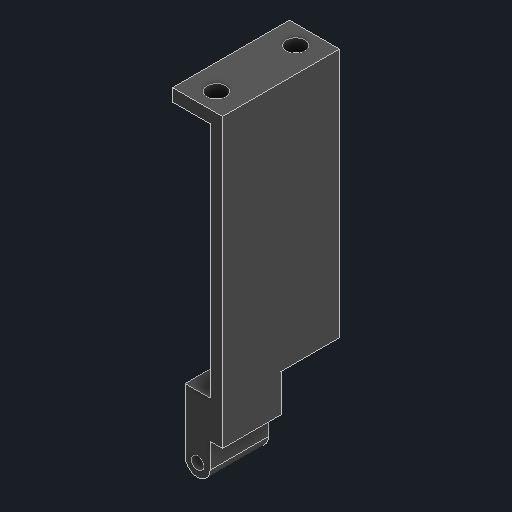
# Autodesk Inventor part: rudder_base
Saved by Autodesk Inventor 2022.2 (Build 262287010, 287A)
## iProperties
Created: 2022-03-30
Part Number: rudder_base
Material: Generic
Document SubType Name: Modeling
Designer: kardo
Density: 1 g/cm^3
Appearance: Dark Plastic
Author: kardo
Autodesk Inventor part; units mm, degrees
ref_plane "YZ Plane" through (0, 0, 0) normal (1, 0, 0) x (0, 1, 0)
ref_plane "XZ Plane" through (0, 0, 0) normal (0, 1, 0) x (-1, 0, 0)
ref_plane "XY Plane" through (0, 0, 0) normal (0, 0, 1) x (1, 0, 0)
derived "parameters_powertrain.ipt"
sketch "sk_base" plane through (0, 0, 0) normal (0, 1, 0) x (-1, 0, 0)
  line L0 (13.09, 0) -> (-13.09, 0) construction
  line L1 (0, -3.74) -> (0, 22.44) construction
  point P0 (0, 0)
  point P1 (0, 15.7)
  point P2 (0, 3)
  point P3 (0, 18.7)
  dimension "d13" = 12.7
  dimension "d14" = 3
  dimension "d15" = 3
  constraints: 3 point on line
  measures "d13" distance of point (0, 3) point (0, 15.7)
  measures "d14" distance of point (0, 15.7) point (0, 18.7)
  measures "d15" distance from line of L0 point (0, 3)
sketch "sk_length" plane through (0, 0, 0) normal (0, 0, 1) x (1, 0, 0)
  line L0 (0, -62.4) -> (0, 10.4) construction
  line L1 (-5.6, 0) -> (5.6, 0) construction
  arc A0 (-2, -50) -> (2, -50) centre (0, -50) ccw
  line L2 (-2, -50) -> (-2, -40)
  line L3 (-2, -40) -> (2, -40)
  line L4 (2, -40) -> (2, -2)
  line L5 (2, -2) -> (-4, -2)
  line L6 (-4, -2) -> (-4, 0)
  line L7 (4, 0) -> (4, -46)
  line L8 (-4, 0) -> (4, 0)
  line L9 (2, -46) -> (2, -50)
  line L10 (4, -46) -> (2, -46)
  point P0 (0, 0)
  dimension "d2" = 50
  dimension "d4" = 4
  dimension "d5" = 6
  dimension "d6" = 4
  dimension "d7" = 2
  dimension "d8" = 2
  dimension "d9" = 2
  dimension "d10" = 4
  constraints: 18 end point, 6 parallel, 3 point on line, 2 point on circle, 2 tangent, 1 centre point, 1 coincident, 1 collinear, 1 perpendicular
  measures "d2" distance from line of L1 A0.centre
  measures "d4" distance between parallel lines of L2 L9
  measures "d5" distance between parallel lines of L3 L10
  measures "d6" distance of L9.start L9.end
  measures "d7" distance between parallel lines of L9 L7
  measures "d8" distance between parallel lines of L7 L4
  measures "d9" distance between parallel lines of L1 L5
  measures "d10" distance between parallel lines of L0 L6
extrude "extrude" add sketch "sk_length" along normal up to surface (18.7 mm away)
hole "drill_base" at (0, 0, 3) at (0, 0, 15.7) direction (0, -1, 0) diameter 3 depth 2 tip angle 118
sketch "sk_remove_fin_attach" plane through (-2, -50, 0) normal (-1, 0, 0) x (0, 0, 1)
  line L0 (0, 10) -> (18.7, 10) projected
  line L1 (0, -2) -> (18.7, -2) projected
  line L2 (9.35, 10) -> (9.35, -2)
  line L3 (0, -2) -> (0, 0) projected
  line L4 (0, -2) -> (0, 10)
  point P0 (0, 50)
  constraints: 4 end point, 2 midpoint
extrude "remove_fin_attach" cut sketch "sk_remove_fin_attach" along normal through all both and the other way through all
hole "drill_fin" at (0, -50, 0) direction (0, 0, 1) diameter 2 end through all both
equation "\"d13\" = rudder_drill_distance"
equation "\"d2\" = rudder_joint_offset_back"
equation "\"rudder_joint_offset_back\" = 50"
equation "\"rudder_drill_distance\" = 12.7"
body "Solid1"
